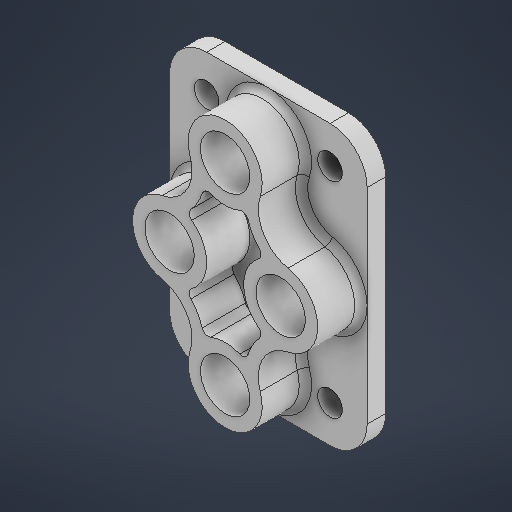
# Autodesk Inventor part: DP807
Saved by Autodesk Inventor 2025.4 (Build 294407000, 407)
## iProperties
Created: 2026-05-07
Part Number: DP807
Material: Generic
Document SubType Name: Modeling
Designer: VuQuan
Density: 1 g/cm^3
Appearance: Default
Author: VuQuan
Autodesk Inventor part; units mm, degrees
ref_plane "YZ Plane" through (0, 0, 0) normal (1, 0, 0) x (0, 1, 0)
ref_plane "XZ Plane" through (0, 0, 0) normal (0, 1, 0) x (-1, 0, 0)
ref_plane "XY Plane" through (0, 0, 0) normal (0, 0, 1) x (1, 0, 0)
sketch "Sketch1" plane through (0, 0, 0) normal (0, 0, 1) x (1, 0, 0)
  line L0 (-25, -56.5) -> (25, -56.5)
  line L1 (40, -41.5) -> (40, 41.5)
  line L2 (25, 56.5) -> (-25, 56.5)
  line L3 (-40, 41.5) -> (-40, -41.5)
  arc A0 (40, 41.5) -> (25, 56.5) centre (25, 41.5) ccw
  arc A1 (25, -56.5) -> (40, -41.5) centre (25, -41.5) ccw
  arc A2 (-40, -41.5) -> (-25, -56.5) centre (-25, -41.5) ccw
  arc A3 (-25, 56.5) -> (-40, 41.5) centre (-25, 41.5) ccw
  circle A4 centre (25, 41.5) radius 5
  circle A5 centre (25, -41.5) radius 5
  circle A6 centre (-25, -41.5) radius 5
  circle A7 centre (-25, 41.5) radius 5
  point P0 (0, 0)
  point P1 (0, 56.5)
  point P2 (40, 0)
  dimension "d0" = 113
  dimension "d1" = 80
  dimension "d2" = 15
  dimension "d3" = 10
  constraints: 8 centre point, 8 end point, 8 point on circle, 8 tangent, 6 equal radius, 4 coincident, 2 midpoint, 2 parallel, 1 horizontal, 1 horizontal alignment, 1 perpendicular, 1 vertical alignment
  measures "d0" distance between parallel lines of L2 L0
  measures "d1" distance between parallel lines of L1 L3
  measures "d2" radius of A0
  measures "d3" diameter of A4
extrude "Extrusion1" add sketch "Sketch1" along normal blind 7.5
sketch "Sketch2" plane through (0, 0, 7.5) normal (0, 0, 1) x (1, 0, 0)
  line L0 (40, -41.5) -> (40, 41.5) projected
  line L1 (25, 56.5) -> (-25, 56.5) projected
  circle A0 centre (0, 39) radius 10
  arc A1 (14.2128, 34.2045) -> (-14.2128, 34.2045) centre (0, 39) ccw
  arc A2 (14.2128, 34.2045) -> (25.4628, 14.7045) centre (28.4256, 29.409) ccw
  arc A3 (25.4628, -14.7045) -> (25.4628, 14.7045) centre (22.5, 0) ccw
  circle A4 centre (22.5, 0) radius 10
  arc A5 (-5.9008, 25.2094) -> (5.9008, 25.2094) centre (0, 39) ccw
  arc A6 (9.2778, 23.633) -> (13.8407, 15.7238) centre (28.4256, 29.409) ccw
  arc A7 (13.5151, 12.0113) -> (13.5151, -12.0113) centre (22.5, 0) ccw
  arc A8 (9.2778, 23.633) -> (5.9008, 25.2094) centre (6.8843, 22.911) ccw
  arc A9 (13.5151, 12.0113) -> (13.8407, 15.7238) centre (12.0176, 14.0132) ccw
  arc A10 (-5.9008, 25.2094) -> (-9.2778, 23.633) centre (-6.8843, 22.911) ccw
  arc A11 (25.4628, -14.7045) -> (14.2128, -34.2045) centre (28.4256, -29.409) ccw
  arc A12 (-14.2128, -34.2045) -> (14.2128, -34.2045) centre (0, -39) ccw
  circle A13 centre (0, -39) radius 10
  arc A14 (-14.2128, -34.2045) -> (-25.4628, -14.7045) centre (-28.4256, -29.409) ccw
  arc A15 (-25.4628, 14.7045) -> (-25.4628, -14.7045) centre (-22.5, 0) ccw
  circle A16 centre (-22.5, 0) radius 10
  arc A17 (-25.4628, 14.7045) -> (-14.2128, 34.2045) centre (-28.4256, 29.409) ccw
  arc A18 (13.8407, -15.7238) -> (13.5151, -12.0113) centre (12.0176, -14.0132) ccw
  arc A19 (13.8407, -15.7238) -> (9.2778, -23.633) centre (28.4256, -29.409) ccw
  arc A20 (5.9008, -25.2094) -> (9.2778, -23.633) centre (6.8843, -22.911) ccw
  arc A21 (-13.8407, 15.7238) -> (-13.5151, 12.0113) centre (-12.0176, 14.0132) ccw
  arc A22 (-13.8407, 15.7238) -> (-9.2778, 23.633) centre (-28.4256, 29.409) ccw
  arc A23 (-13.5151, -12.0113) -> (-13.5151, 12.0113) centre (-22.5, 0) ccw
  arc A24 (-9.2778, -23.633) -> (-13.8407, -15.7238) centre (-28.4256, -29.409) ccw
  arc A25 (-13.5151, -12.0113) -> (-13.8407, -15.7238) centre (-12.0176, -14.0132) ccw
  arc A26 (5.9008, -25.2094) -> (-5.9008, -25.2094) centre (0, -39) ccw
  arc A27 (-9.2778, -23.633) -> (-5.9008, -25.2094) centre (-6.8843, -22.911) ccw
  point P0 (0, 0)
  point P1 (0, 54)
  point P2 (37.5, 0)
  point P3 (0, -54)
  point P4 (-37.5, 0)
  point P5 (0, 0)
  point P6 (9.2778, -23.633)
  dimension "d6" = 20
  dimension "d7" = 15
  dimension "d8" = 2.5
  dimension "d9" = 15
  dimension "d10" = 2.5
  dimension "d11" = 20
  dimension "d12" = 2.5
  dimension "d13" = 5
  dimension "d14" = 5
  dimension "d17" = 360
  dimension "d21" = 360
  constraints: 56 point on circle, 28 centre point, 11 coincident, 10 tangent, 7 equal radius, 3 horizontal alignment, 3 vertical alignment, 92 other
  measures "d6" diameter of A0
  measures "d7" radius of A1
  measures "d8" distance from line of L1 point (0, 54)
  measures "d9" radius of A2
  measures "d10" distance from line of L0 point (37.5, 0)
  measures "d11" radius of A6
  measures "d12" radius of A8
  measures "d13" radial gap between concentric circles of A7 A4
  measures "d14" radial gap between concentric circles of A0 A5
extrude "Extrusion2" add sketch "Sketch2" along normal blind 17.5
fillet "Fillet1" radius 2.5 8 edges at (37.5, 0, 7.5) (15.4328, -21.9131, 7.5) (0, -54, 7.5) (-15.4328, -21.9131, 7.5) (-37.5, 0, 7.5) (-15.4328, 21.9131, 7.5) (0, 54, 7.5) (15.4328, 21.9131, 7.5)
body "Solid1"
